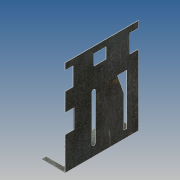
# Autodesk Inventor part: Platina lateral interna 1
Saved by Autodesk Inventor 2016 (Build 200138000, 138)
## iProperties
Created: 2016-05-25
Part Number: Platina lateral interna 1
Material: Steel
Document SubType Name: Modeling
Designer: Familia
Density: 7.85 g/cm^3
Appearance: Plate
Mass: 52.6189 g
Surface Area: 274.145 cm^2
Volume: 6.70305 cm^3
Author: Familia
Autodesk Inventor part; units mm, degrees
ref_plane "YZ Plane" through (0, 0, 0) normal (1, 0, 0) x (0, 1, 0)
ref_plane "XZ Plane" through (0, 0, 0) normal (0, 1, 0) x (-1, 0, 0)
ref_plane "XY Plane" through (0, 0, 0) normal (0, 0, 1) x (1, 0, 0)
sketch "Sketch1" plane through (0, 0, 0) normal (0, 1, 0) x (-1, 0, 0)
  line L0 (0, 0) -> (0, 130)
  line L1 (0, 130) -> (0.5, 130)
  line L2 (0.5, 130) -> (0.5, 0.5)
  line L3 (0.5, 0.5) -> (32, 0.5)
  line L4 (32, 0.5) -> (32, 0)
  line L5 (32, 0) -> (0, 0)
  dimension "d0" = 0.5
  dimension "d1" = 130
  dimension "d2" = 32
  constraints: 12 end point, 6 perpendicular, 1 vertical
  measures "d0" distance of L0.end L1.end
  measures "d1" distance of L0.start L0.end
  measures "d2" distance between parallel lines of L4 L0
extrude "Extrusion1" add sketch "Sketch1" along normal mid plane 100
sketch "Sketch2" plane through (0, -50, 0) normal (1, 0, 0) x (0, 0, -1)
  line L0 (-121.2604, 39.005) -> (-106.3744, 39.005)
  line L1 (-106.3744, 39.005) -> (-106.3744, 56.2727)
  line L2 (-106.3744, 56.2727) -> (-121.2604, 56.2727)
  line L3 (-121.2604, 56.2727) -> (-121.2604, 39.005)
  line L4 (-121.2604, -4.0598) -> (-96.0852, -4.0598)
  line L5 (-96.0852, -4.0598) -> (-96.0852, 11.0828)
  line L6 (-96.0852, 11.0828) -> (-121.2604, 11.0828)
  line L7 (-121.2604, 11.0828) -> (-121.2604, -4.0598)
  line L8 (-71.2006, -4.0598) -> (-44.9947, -4.0598)
  line L9 (-44.9947, -4.0598) -> (-44.9947, 12.1839)
  line L10 (-44.9947, 12.1839) -> (-71.2006, 12.1839)
  line L11 (-71.2006, 12.1839) -> (-71.2006, -4.0598)
  line L12 (-121.2604, 102.7324) -> (-96.0852, 102.7324)
  line L13 (-96.0852, 102.7324) -> (-96.0852, 88.3791)
  line L14 (-96.0852, 88.3791) -> (-121.2604, 88.3791)
  line L15 (-121.2604, 88.3791) -> (-121.2604, 102.7324)
  line L16 (-15.0452, 39.005) -> (-76.9263, 39.005) construction
  line L17 (-15.0452, 41.4826) -> (-76.9263, 41.4826)
  line L18 (-76.9263, 36.5275) -> (-15.0452, 36.5275)
  arc A0 (-15.0452, 36.5275) -> (-15.0452, 41.4826) centre (-15.0452, 39.005) ccw
  arc A1 (-76.9263, 41.4826) -> (-76.9263, 36.5275) centre (-76.9263, 39.005) ccw
  line L19 (-79.4038, 71.4223) -> (-79.4038, 84.1949)
  line L20 (-79.4038, 84.1949) -> (-10.4206, 84.1949)
  line L21 (-10.4206, 84.1949) -> (-10.4206, 80.231)
  line L22 (-10.4206, 80.231) -> (-54.0237, 80.231)
  line L23 (-54.0237, 80.231) -> (-79.4038, 71.4223)
  point P0 (0, 50)
  point P1 (-45.9857, 39.005)
  constraints: 50 end point, 9 parallel, 7 perpendicular, 5 horizontal, 4 point on circle, 4 tangent, 3 point on line, 2 centre point, 1 midpoint, 1 vertical
extrude "Extrusion2" cut sketch "Sketch2" against normal blind 100
sketch "Sketch3" plane through (-32, 50, 0.5) normal (0, 0, 1) x (1, 0, 0)
  line L0 (5, -15) -> (25, -15) construction
  line L1 (5, -16.75) -> (25, -16.75)
  line L2 (25, -13.25) -> (5, -13.25)
  arc A0 (5, -13.25) -> (5, -16.75) centre (5, -15) ccw
  arc A1 (25, -16.75) -> (25, -13.25) centre (25, -15) ccw
  line L3 (5, -20) -> (25, -20) construction
  line L4 (5, -21.75) -> (25, -21.75)
  line L5 (25, -18.25) -> (5, -18.25)
  arc A2 (5, -18.25) -> (5, -21.75) centre (5, -20) ccw
  arc A3 (25, -21.75) -> (25, -18.25) centre (25, -20) ccw
  line L6 (5, -25) -> (25, -25) construction
  line L7 (5, -26.75) -> (25, -26.75)
  line L8 (25, -23.25) -> (5, -23.25)
  arc A4 (5, -23.25) -> (5, -26.75) centre (5, -25) ccw
  arc A5 (25, -26.75) -> (25, -23.25) centre (25, -25) ccw
  line L9 (5, -30) -> (25, -30) construction
  line L10 (5, -31.75) -> (25, -31.75)
  line L11 (25, -28.25) -> (5, -28.25)
  arc A6 (5, -28.25) -> (5, -31.75) centre (5, -30) ccw
  arc A7 (25, -31.75) -> (25, -28.25) centre (25, -30) ccw
  line L12 (15, -15) -> (15, -20)
  line L13 (15, -20) -> (15, -25)
  line L14 (15, -25) -> (15, -30)
  line L15 (0, 0) -> (0, -100) projected
  line L16 (0, 0) -> (31.5, 0) projected
  point P0 (32, -50)
  dimension "d7" = 1.75
  dimension "d8" = 15
  dimension "d9" = 20
  dimension "d10" = 15
  dimension "d11" = 5
  constraints: 38 end point, 16 point on circle, 16 tangent, 8 centre point, 7 parallel, 4 midpoint, 3 equal radius, 3 vertical alignment, 2 collinear, 2 perpendicular, 1 horizontal, 1 vertical
  measures "d7" radius of A0
  measures "d8" distance between parallel lines of L12 L15
  measures "d9" distance of L0.start L0.end
  measures "d10" distance between parallel lines of L0 L16
  measures "d11" distance between parallel lines of L0 L3
extrude "Extrusion3" cut sketch "Sketch3" against normal blind 100
sketch "Sketch4" plane through (-32, 50, 0.5) normal (0, 0, 1) x (1, 0, 0)
  line L0 (-3.8096, -70.3357) -> (24.0538, -70.3357)
  line L1 (24.0538, -70.3357) -> (24.0538, -93.8822)
  line L2 (24.0538, -93.8822) -> (-3.8096, -93.8822)
  line L3 (-3.8096, -93.8822) -> (-3.8096, -70.3357)
  point P0 (32, -50)
  constraints: 8 end point, 2 parallel, 1 horizontal, 1 perpendicular
extrude "Extrusion4" cut sketch "Sketch4" against normal through all
body "Solid1"
